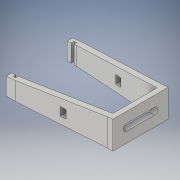
# Autodesk Inventor part: holder
Saved by Autodesk Inventor 2019 (Build 230136000, 136)
## iProperties
Created: 2019-01-14
Part Number: holder
Material: Generic
Document SubType Name: Modeling
Designer: erwin
Density: 1 g/cm^3
Appearance: Default
Author: erwin
Autodesk Inventor part; units mm, degrees
ref_plane "YZ Plane" through (0, 0, 0) normal (1, 0, 0) x (0, 1, 0)
ref_plane "XZ Plane" through (0, 0, 0) normal (0, 1, 0) x (-1, 0, 0)
ref_plane "XY Plane" through (0, 0, 0) normal (0, 0, 1) x (1, 0, 0)
sketch "Sketch1" plane through (0, 0, 0) normal (0, 1, 0) x (-1, 0, 0)
  line L0 (-0.5, 11) -> (0.5, 11) construction
  line L1 (0.5, 11) -> (0.5, -11) construction
  line L2 (0.5, -11) -> (-0.5, -11) construction
  line L3 (-0.5, -11) -> (-0.5, 11) construction
  line L4 (-0.5, 11) -> (0.5, -11) construction
  line L5 (0.5, 11) -> (-0.5, -11) construction
  line L6 (-0.5, 11) -> (-0.5, 9.9373) construction
  line L7 (-1.5, 10) -> (-1.5, 12)
  line L8 (-1.5, 12) -> (1.5, 12)
  line L9 (1.5, 12) -> (1.5, 10)
  line L10 (1.5, 10) -> (-1.5, 12) construction
  line L11 (-1.5, 10) -> (1.5, 12) construction
  line L12 (-0.5, 11) -> (0.5, 11)
  line L13 (0.5, 11) -> (0.5, 10)
  line L14 (-0.5, 10) -> (-0.5, 11)
  line L15 (1.5, 10) -> (0.5, 10)
  line L16 (-0.5, 10) -> (-1.5, 10)
  line L17 (-34.5, 0) -> (-32.5, 0)
  line L18 (-32.5, 0) -> (-32.5, 10)
  line L19 (-32.5, 10) -> (-34.5, 10)
  line L20 (-34.5, 10) -> (-34.5, 0)
  line L21 (-32.5, 10) -> (-1.5, 12)
  line L22 (-1.5, 10) -> (-32.5, 8)
  point P0 (0, 0)
  point P1 (0, 11)
  dimension "d0" = 1
  dimension "d1" = 22
  dimension "d2" = 3
  dimension "d3" = 2
  dimension "d4" = 2
  dimension "d5" = 10
  dimension "d6" = 35
  constraints: 46 end point, 9 parallel, 5 horizontal, 5 midpoint, 5 perpendicular, 3 point on line
  measures "d0" distance of L1.end L2.end
  measures "d1" distance of L0.end L1.end
  measures "d2" distance of L7.end L8.end
  measures "d3" distance of L7.start L7.end
  measures "d4" distance of L19.end L18.end
  measures "d5" distance of L18.end L17.end
  measures "d6" distance between parallel lines of L1 L20
extrude "Extrusion1" add sketch "Sketch1" along normal blind 10
mirror "Mirror1" about plane through (34.5, 0, 0) normal (0, 0, -1) of "Extrusion1"
draft "FaceDraft1" angle 6 pull direction (-1, 0, 0) faces at (11.8333, 10, -10.6667) fixed edges at (34.5, 10, 0)
sketch "Sketch2" plane through (1.5, 0, -12) normal (0, 0, -1) x (-1, 0, 0)
  line L0 (-15, 5.5) -> (-17, 5.5)
  line L1 (-17, 5.5) -> (-17, 2.5)
  line L2 (-17, 2.5) -> (-15, 2.5)
  line L3 (-15, 2.5) -> (-15, 5.5)
  line L4 (-15, 5.5) -> (-17, 2.5) construction
  line L5 (-17, 5.5) -> (-15, 2.5) construction
  line L6 (0, 0) -> (-31, 0) projected
  line L7 (3, 0) -> (3, 6.2162) projected
  point P0 (1.5, 0)
  point P1 (-16, 4)
  dimension "d10" = 2
  dimension "d11" = 3
  dimension "d12" = 2.5
  dimension "d13" = 18
  constraints: 12 end point, 2 midpoint, 2 parallel, 1 horizontal, 1 perpendicular
  measures "d10" distance of L2.end L1.end
  measures "d11" distance of L1.end L0.end
  measures "d12" distance between parallel lines of L6 L2
  measures "d13" distance between parallel lines of L7 L3
extrude "Extrusion2" cut sketch "Sketch2" against normal through all
sketch "Sketch3" plane through (32.5, 0, -8) normal (-1, 0, 0) x (0, 0, 1)
  line L0 (13, 5) -> (3, 5) construction
  line L1 (13, 6.25) -> (3, 6.25)
  line L2 (3, 3.75) -> (13, 3.75)
  arc A0 (13, 3.75) -> (13, 6.25) centre (13, 5) ccw
  arc A1 (3, 6.25) -> (3, 3.75) centre (3, 5) ccw
  point P0 (8, 0)
  point P1 (8, 5)
  dimension "d16" = 5
  dimension "d17" = 2.5
  constraints: 8 end point, 4 point on circle, 4 tangent, 2 centre point, 1 horizontal, 1 midpoint, 1 parallel
  measures "d16" distance of point (8, 5) L0.end
  measures "d17" diameter of A1
extrude "Extrusion3" cut sketch "Sketch3" against normal through all
move faces "Move1" translate (-0.5, 0, 0) faces at (-1.5, 4.1442, -11.3333) (-1.5, 4.1442, 11.3333)
body "Solid1"
